Autodesk Fusion 360 part; units mm, degrees
(part 9 of 9)
equation "d2492 = ( FootHeight ) + PanHeight - DeckThick"
equation "d2494 = ( BaseX + LeftRun + FaucetGap + ( RightRun + ModuleGap ) / 2 ) + ( ( ( ( RightRun - ModuleGap ) / 2 ) - Wall - 2 mm ) - DeckClearance )"
equation "d2495 = ( BaseY ) + ( 10 mm - DeckClearance )"
equation "d2496 = 2 mm + 2 * DeckClearance"
equation "d2497 = 5 mm + 2 * DeckClearance"
equation "d2498 = DeckThick"
equation "d2500 = FootHeight"
equation "d2502 = ( BaseX + LeftRun + FaucetGap + ( RightRun + ModuleGap ) / 2 ) + ( ( ( RightRun - ModuleGap ) / 2 ) - Wall - 2 mm )"
equation "d2503 = ( BaseY ) + ( 10 mm )"
equation "d2506 = PanHeight"
equation "d2508 = ( FootHeight ) - 0.2 mm"
equation "d2510 = ( BaseX ) + ( LeftSideDepth )"
equation "d2511 = ( BaseY + Depth + ModuleGap ) + ( ( LeftReach ) - ( ( -1 mm ) + ( ( LeftReach ) + 2 mm ) ) )"
equation "d2512 = DrainExtension + 2 mm"
equation "d2513 = ( LeftReach ) + 2 mm"
equation "d2514 = PanHeight + 0.4 mm"
equation "d2516 = ( BaseY + Depth + ModuleGap ) + ( ( LeftReach ) - ( Wall ) )"
equation "d2518 = ( ( BaseX ) + ( ( LeftSideDepth ) - Wall - 0.1 mm ) )"
equation "d2519 = -( -( ( FootHeight ) + FloorMin + DrainExtension * tan(DrainSlope) + ( ( LeftSideDepth ) - ( ( LeftSideDepth ) - Wall - 0.1 mm ) ) * tan(DrainSlope) ) )"
equation "d2520 = ( ( BaseX ) + ( ( LeftSideDepth ) + 1 mm ) )"
equation "d2521 = -( -( ( FootHeight ) + FloorMin + DrainExtension * tan(DrainSlope) + ( ( LeftSideDepth ) - ( ( LeftSideDepth ) + 1 mm ) ) * tan(DrainSlope) ) )"
equation "d2522 = -( -( ( FootHeight ) + PanHeight + 1 mm ) )"
equation "d2523 = -( -( -( ( LeftReach ) - 2 * Wall ) ) )"
equation "d2525 = ( FootHeight ) + PanHeight - DeckThick"
equation "d2527 = ( BaseX ) + ( 10 mm - DeckClearance )"
equation "d2528 = ( BaseY + Depth + ModuleGap ) + ( ( LeftReach ) - ( ( ( Wall ) - DeckClearance ) + ( 2 mm + 2 * DeckClearance ) ) )"
equation "d2529 = 5 mm + 2 * DeckClearance"
equation "d2530 = 2 mm + 2 * DeckClearance"
equation "d2531 = DeckThick"
equation "d2533 = FootHeight"
equation "d2535 = ( BaseX ) + ( 10 mm )"
equation "d2536 = ( BaseY + Depth + ModuleGap ) + ( ( LeftReach ) - ( ( Wall ) + ( 2 mm ) ) )"
equation "d2539 = PanHeight"
equation "d2541 = ( FootHeight ) + PanHeight - DeckThick"
equation "d2543 = ( BaseX ) + ( 10 mm - DeckClearance )"
equation "d2544 = ( BaseY + Depth + ModuleGap ) + ( ( LeftReach ) - ( ( ( ( LeftReach ) - Wall - 2 mm ) - DeckClearance ) + ( 2 mm + 2 * DeckClearance ) ) )"
equation "d2545 = 5 mm + 2 * DeckClearance"
equation "d2546 = 2 mm + 2 * DeckClearance"
equation "d2547 = DeckThick"
equation "d2549 = FootHeight"
equation "d2551 = ( BaseX ) + ( 10 mm )"
equation "d2552 = ( BaseY + Depth + ModuleGap ) + ( ( LeftReach ) - ( ( ( LeftReach ) - Wall - 2 mm ) + ( 2 mm ) ) )"
equation "d2555 = PanHeight"
equation "d2557 = ( FootHeight ) - 0.2 mm"
equation "d2559 = ( BaseX + LeftRun + FaucetGap + RightRun - RightSideDepth ) + ( ( RightSideDepth ) - ( ( RightSideDepth ) + ( DrainExtension + 2 mm ) ) )"
equation "d2560 = ( BaseY + Depth + ModuleGap ) + ( -1 mm )"
equation "d2561 = DrainExtension + 2 mm"
equation "d2562 = ( RightReach ) + 2 mm"
equation "d2563 = PanHeight + 0.4 mm"
equation "d2565 = ( BaseY + Depth + ModuleGap ) + ( Wall )"
equation "d2567 = ( ( BaseX + LeftRun + FaucetGap + RightRun - RightSideDepth ) + ( ( RightSideDepth ) - ( ( RightSideDepth ) - Wall - 0.1 mm ) ) )"
equation "d2568 = -( -( ( FootHeight ) + FloorMin + DrainExtension * tan(DrainSlope) + ( ( RightSideDepth ) - ( ( RightSideDepth ) - Wall - 0.1 mm ) ) * tan(DrainSlope) ) )"
equation "d2569 = ( ( BaseX + LeftRun + FaucetGap + RightRun - RightSideDepth ) + ( ( RightSideDepth ) - ( ( RightSideDepth ) + 1 mm ) ) )"
equation "d2570 = -( -( ( FootHeight ) + FloorMin + DrainExtension * tan(DrainSlope) + ( ( RightSideDepth ) - ( ( RightSideDepth ) + 1 mm ) ) * tan(DrainSlope) ) )"
equation "d2571 = -( -( ( FootHeight ) + PanHeight + 1 mm ) )"
equation "d2572 = ( RightReach ) - 2 * Wall"
equation "d2574 = ( FootHeight ) + PanHeight - DeckThick"
equation "d2576 = ( BaseX + LeftRun + FaucetGap + RightRun - RightSideDepth ) + ( ( RightSideDepth ) - ( ( 10 mm - DeckClearance ) + ( 5 mm + 2 * DeckClearance ) ) )"
equation "d2577 = ( BaseY + Depth + ModuleGap ) + ( ( Wall ) - DeckClearance )"
equation "d2578 = 5 mm + 2 * DeckClearance"
equation "d2579 = 2 mm + 2 * DeckClearance"
equation "d2580 = DeckThick"
equation "d2582 = FootHeight"
equation "d2584 = ( BaseX + LeftRun + FaucetGap + RightRun - RightSideDepth ) + ( ( RightSideDepth ) - ( ( 10 mm ) + ( 5 mm ) ) )"
equation "d2585 = ( BaseY + Depth + ModuleGap ) + ( Wall )"
equation "d2588 = PanHeight"
equation "d2590 = ( FootHeight ) + PanHeight - DeckThick"
equation "d2592 = ( BaseX + LeftRun + FaucetGap + RightRun - RightSideDepth ) + ( ( RightSideDepth ) - ( ( 10 mm - DeckClearance ) + ( 5 mm + 2 * DeckClearance ) ) )"
equation "d2593 = ( BaseY + Depth + ModuleGap ) + ( ( ( RightReach ) - Wall - 2 mm ) - DeckClearance )"
equation "d2594 = 5 mm + 2 * DeckClearance"
equation "d2595 = 2 mm + 2 * DeckClearance"
equation "d2596 = DeckThick"
equation "d2598 = FootHeight"
equation "d2600 = ( BaseX + LeftRun + FaucetGap + RightRun - RightSideDepth ) + ( ( RightSideDepth ) - ( ( 10 mm ) + ( 5 mm ) ) )"
equation "d2601 = ( BaseY + Depth + ModuleGap ) + ( ( RightReach ) - Wall - 2 mm )"
equation "d2604 = PanHeight"
equation "d2606 = ( UpperDeckHeight - PanHeight ) - 0.2 mm"
equation "d2608 = ( BaseX ) + ( -1 mm )"
equation "d2609 = ( BaseY ) + ( Depth )"
equation "d2610 = ( TowerWidth ) + 2 mm"
equation "d2611 = DrainExtension + 2 mm"
equation "d2612 = PanHeight + 0.4 mm"
equation "d2614 = ( BaseX ) + ( Wall )"
equation "d2616 = -( -( ( UpperDeckHeight - PanHeight ) + FloorMin + DrainExtension * tan(DrainSlope) + ( ( Depth ) - ( ( Depth ) - Wall - 0.1 mm ) ) * tan(DrainSlope) ) )"
equation "d2617 = ( ( BaseY ) + ( ( Depth ) - Wall - 0.1 mm ) )"
equation "d2618 = -( -( ( UpperDeckHeight - PanHeight ) + FloorMin + DrainExtension * tan(DrainSlope) + ( ( Depth ) - ( ( Depth ) + 1 mm ) ) * tan(DrainSlope) ) )"
equation "d2619 = ( ( BaseY ) + ( ( Depth ) + 1 mm ) )"
equation "d2620 = -( -( ( UpperDeckHeight - PanHeight ) + PanHeight + 1 mm ) )"
equation "d2621 = ( TowerWidth ) - 2 * Wall"
equation "d2623 = ( UpperDeckHeight - PanHeight ) + PanHeight - DeckThick"
equation "d2625 = ( BaseX ) + ( ( Wall ) - DeckClearance )"
equation "d2626 = ( BaseY ) + ( 13 mm - DeckClearance )"
equation "d2627 = 2 mm + 2 * DeckClearance"
equation "d2628 = 5 mm + 2 * DeckClearance"
equation "d2629 = DeckThick"
equation "d2631 = UpperDeckHeight - PanHeight"
equation "d2633 = ( BaseX ) + ( Wall )"
equation "d2634 = ( BaseY ) + ( 13 mm )"
equation "d2637 = PanHeight"
equation "d2639 = ( UpperDeckHeight - PanHeight ) + PanHeight - DeckThick"
equation "d2641 = ( BaseX ) + ( ( ( TowerWidth ) - Wall - 2 mm ) - DeckClearance )"
equation "d2642 = ( BaseY ) + ( 13 mm - DeckClearance )"
equation "d2643 = 2 mm + 2 * DeckClearance"
equation "d2644 = 5 mm + 2 * DeckClearance"
equation "d2645 = DeckThick"
equation "d2647 = UpperDeckHeight - PanHeight"
equation "d2649 = ( BaseX ) + ( ( TowerWidth ) - Wall - 2 mm )"
equation "d2650 = ( BaseY ) + ( 13 mm )"
equation "d2653 = PanHeight"
named bodies: "L1_DrainPan", "L1_RemovableGrate", "L1_Foot_00", "L1_Foot_01", "L1_Foot_10", "L1_Foot_11", "L2_DrainPan", "L2_RemovableGrate", "L2_Foot_00", "L2_Foot_01", "L2_Foot_10", "L2_Foot_11", "R1_DrainPan", "R1_RemovableGrate", "R1_Foot_00", "R1_Foot_01", "R1_Foot_10", "R1_Foot_11", "R2_DrainPan", "R2_RemovableGrate", "R2_Foot_00", "R2_Foot_01", "R2_Foot_10", "R2_Foot_11", "LS_DrainPan", "LS_RemovableGrate", "LS_Foot_00", "LS_Foot_01", "LS_Foot_10", "LS_Foot_11", "RS_DrainPan", "RS_RemovableGrate", "RS_Foot_00", "RS_Foot_01", "RS_Foot_10", "RS_Foot_11", "UP_DrainPan", "UP_RemovableGrate", "Tower_SideFrame_1", "Tower_SideFrame_2", "FIT_Tight", "FIT_Nominal", "FIT_Loose"
